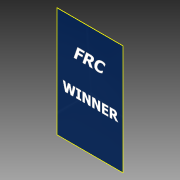
# Autodesk Inventor part: Winner Banner
Saved by Autodesk Inventor 2014 (Build 180170000, 170)
## iProperties
Created: 2015-04-18
Part Number: Winner Banner
Material: Generic
Document SubType Name: Modeling
Designer: Gus
Density: 1 g/cm^3
Appearance: Default
Author: Gus
Autodesk Inventor part; units mm, degrees
ref_plane "YZ Plane" through (0, 0, 0) normal (1, 0, 0) x (0, 1, 0)
ref_plane "XZ Plane" through (0, 0, 0) normal (0, 1, 0) x (-1, 0, 0)
ref_plane "XY Plane" through (0, 0, 0) normal (0, 0, 1) x (1, 0, 0)
sketch "Sketch1" plane through (0, 0, 0) normal (0, 0, 1) x (1, 0, 0)
  line L0 (0, 0) -> (914.4, 0)
  line L1 (914.4, 0) -> (914.4, 1524)
  line L2 (914.4, 1524) -> (0, 1524)
  line L3 (0, 1524) -> (0, 0)
  dimension "d0" = 914.4
  dimension "d1" = 1524
  constraints: 8 end point, 2 parallel, 1 horizontal, 1 perpendicular
  measures "d0" distance of L2.end L1.end
  measures "d1" distance of L1.end L0.end
extrude "Extrusion1" add sketch "Sketch1" along normal blind 5.08
sketch "Sketch2" plane through (0, 0, 5.08) normal (0, 0, 1) x (1, 0, 0)
  line L0 (0, 0) -> (914.4, 0) projected
  line L1 (914.4, 0) -> (914.4, 1524) projected
  line L2 (914.4, 1524) -> (0, 1524) projected
  line L3 (0, 1524) -> (0, 0) projected
  line L4 (218.9125, 1195.0171) -> (654.4999, 1195.0171) construction
  line L5 (654.4999, 1195.0171) -> (654.4999, 1036.689) construction
  line L6 (654.4999, 1036.689) -> (218.9125, 1036.689) construction
  line L7 (218.9125, 1036.689) -> (218.9125, 1195.0171) construction
  line L8 (80.552, 697.9442) -> (847.9037, 697.9442) construction
  line L9 (847.9037, 697.9442) -> (847.9037, 570.9442) construction
  line L10 (847.9037, 570.9442) -> (80.552, 570.9442) construction
  line L11 (80.552, 570.9442) -> (80.552, 697.9442) construction
  constraints: 4 other
body "Solid1"
